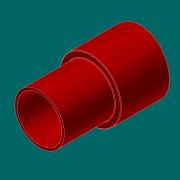
# Autodesk Inventor part: A1-19027-400-12 HCWI liner - port
Saved by Autodesk Inventor 2017.3 (Build 213257000, 257)
## iProperties
Created: 2019-08-16
Part Number: A1-19027-400-12 HCWI liner - port
Material: Iron, HCWI
Document SubType Name: Modeling
Designer: GVD
Density: 7.33517 g/cm^3
Appearance: Iron Gray(1)
Mass: 1703.64 g
Surface Area: 717.946 cm^2
Volume: 232.257 cm^3
Description: 2 19/32" ID x 1/2" WALL x 5 7/8" HCWI LINER, ASTM A532 CLASS III TYPE A, PF#(TBD)
Author: GVD
Autodesk Inventor part; units mm, degrees
ref_plane "YZ Plane" through (0, 0, 0) normal (1, 0, 0) x (0, 1, 0)
ref_plane "XZ Plane" through (0, 0, 0) normal (0, 1, 0) x (-1, 0, 0)
ref_plane "XY Plane" through (0, 0, 0) normal (0, 0, 1) x (1, 0, 0)
sketch "Sketch1" plane through (0, 0, 0) normal (0, 0, 1) x (1, 0, 0)
  circle A0 centre (0, 0) radius 36.576
  circle A1 centre (0, 0) radius 33
  circle A2 centre (0, 0) radius 45.2437
  dimension "d0" = 73.152
  dimension "d1" = 66
  dimension "d11" = 90.4875
  constraints: 3 centre point, 3 coincident
  measures "d0" diameter of A0
  measures "d1" diameter of A1
  measures "d11" diameter of A2
extrude "Extrusion1" add sketch "Sketch1" along normal blind 539.75 contours A0
extrude "Extrusion4" add sketch "Sketch1" along normal blind 465.1375 contours A2
sketch "Sketch3" plane through (0, 0, 0) normal (1, 0, 0) x (0, 1, 0)
  circle A0 centre (0, 0) radius 393.7
  dimension "d7" = 787.4
  constraints: 1 centre point, 1 coincident
  measures "d7" diameter of A0
extrude "Extrusion3" cut sketch "Sketch3" along normal through all both and the other way through all
fillet "Fillet2" radius 0.7937 1 edges at (-36.576, 0, 465.1375)
chamfer "Chamfer2" distance 0.7937 angle 45 1 edges at (-45.2437, 0, 465.1375)
body "Solid1"
